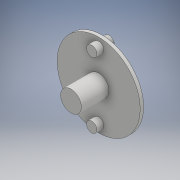
# Autodesk Inventor part: EE Wheel
Saved by Autodesk Inventor 2017 (Build 210142000, 142)
## iProperties
Created: 2018-10-18
Part Number: EE Wheel
Material: Generic
Document SubType Name: Modeling
Designer: Cameron
Density: 1 g/cm^3
Appearance: Default
Author: Cameron
Autodesk Inventor part; units mm, degrees
ref_plane "YZ Plane" through (0, 0, 0) normal (1, 0, 0) x (0, 1, 0)
ref_plane "XZ Plane" through (0, 0, 0) normal (0, 1, 0) x (-1, 0, 0)
ref_plane "XY Plane" through (0, 0, 0) normal (0, 0, 1) x (1, 0, 0)
sketch "Sketch1" plane through (0, 0, 0) normal (0, 1, 0) x (-1, 0, 0)
  circle A0 centre (0, 0) radius 3
  dimension "d0" = 6
  constraints: 1 centre point, 1 coincident
  measures "d0" diameter of A0
extrude "Extrusion1" add sketch "Sketch1" along normal blind 6
sketch "Sketch2" plane through (0, 6, 0) normal (0, 1, 0) x (1, 0, 0)
  circle A0 centre (0, 0) radius 3 projected
  circle A1 centre (0, 0) radius 12
  dimension "d3" = 24
  constraints: 1 centre point, 1 coincident
  measures "d3" diameter of A1
extrude "Extrusion2" add sketch "Sketch2" along normal blind 1 contours A0 | A1
sketch "Sketch3" plane through (0, 7, 0) normal (0, 1, 0) x (1, 0, 0)
  circle A0 centre (0, 0) radius 12 projected
  line L0 (0, 0) -> (0, -9.5)
  line L1 (0, -9.5) -> (0, 9.5)
  circle A1 centre (0, -9.5) radius 1.5
  circle A2 centre (0, 9.5) radius 1.5
  dimension "d6" = 9.5
  dimension "d7" = 19
  dimension "d8" = 3
  dimension "d9" = 3
  constraints: 4 end point, 2 centre point, 2 coincident, 1 point on line, 1 vertical
  measures "d6" distance of L0.start L0.end
  measures "d7" distance of L0.end L1.end
  measures "d8" diameter of A1
  measures "d9" diameter of A2
extrude "Extrusion3" add sketch "Sketch3" along normal blind 2 and the other way blind 3 contours A1 | A2
sketch "Sketch4" plane through (0, 0, 0) normal (0, -1, 0) x (1, 0, 0)
  circle A0 centre (0, 0) radius 3 projected
extrude "Extrusion4" add sketch "Sketch4" along normal blind 2
body "Solid1"
